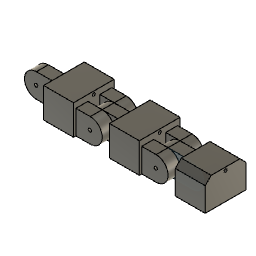
Complete Finger v1 (Autodesk Fusion 360 design; units mm, degrees)
Autodesk Fusion 360 part; units mm, degrees
sketch "Sketch3" plane through (0, 0, 0) normal (0, 1, 0) x (1, 0, 0)
  circle A0 centre (10, -10) radius 10
  circle A1 centre (-12.5, -10) radius 10
sketch "Sketch4" plane through (0, 0, 0) normal (0, 1, 0) x (1, 0, 0)
  line L0 (10, -20) -> (30, -20)
  line L1 (30, -20) -> (30, 0)
  line L2 (30, 0) -> (10, 0)
  line L3 (10, 0) -> (10, -20)
  circle A0 centre (30, -10) radius 10
  constraint horizontal L0
  constraint perpendicular L0 L1
  constraint perpendicular L1 L2
  constraint perpendicular L2 L3
  constraint midpoint L1 A0.centre
  constraint coincident L1.end A0
extrude "Extrude2" add sketch "Sketch4" sketch "Sketch3" along normal blind 10 of sketch 2 makes body 1 at (-2.5124, 6.6667, 10.4985) makes body 2 at (23.3333, 0, 13.3333)
sketch "Sketch5" plane through (0, 0, 0) normal (0, -1, 0) x (1, 0, 0)
  circle A0 centre (-12.5, 10) radius 10
  circle A1 centre (-12.5, 10) radius 10
  circle A2 centre (10, 10) radius 10
  line L0 (-12.5, 20) -> (10, 20)
  line L1 (10, 10) -> (10, 0)
  line L2 (-12.5, 0) -> (-12.5, 20)
  line L3 (10, 20) -> (10, 10)
  line L4 (-12.5, 0) -> (10, 0)
  constraint concentric A0 A1
  constraint coincident A1 L0.start
  constraint tangent A1 L0
  constraint horizontal L0
  constraint coincident A2.centre L1.start
  constraint coincident A2 L1.end
  constraint perpendicular L0 L1
  constraint coincident A1 L2.start
  constraint perpendicular L0 L2
  constraint perpendicular L0 L3
  constraint tangent A2 L4
extrude "Extrude3" add sketch "Sketch5" along normal blind 10 bodies 1 2
sketch "Sketch6" plane through (0, 10, 0) normal (0, 1, 0) x (-1, 0, 0)
  circle A0 centre (12.5, 10) radius 10
  circle A1 centre (12.5, 10) radius 10
  circle A2 centre (-10, 10) radius 10
  line L0 (-10, 20) -> (12.5, 20)
  line L1 (12.5, 10) -> (12.5, 0)
  line L2 (-10, 0) -> (-10, 10)
  line L3 (-10, 10) -> (-10, 20)
  line L4 (12.5, 10) -> (12.5, 20)
  line L5 (-10, 0) -> (12.5, 0)
  constraint concentric A0 A1
  constraint coincident A2 L0.start
  constraint coincident A1 L0.end
  constraint tangent A1 L0
  constraint horizontal L0
  constraint coincident A0.centre A1.centre
  constraint coincident A1 L1.end
  constraint perpendicular L0 L1
  constraint coincident A2 L2.start
  constraint coincident A2.centre L2.end
  constraint parallel L1 L2
  constraint perpendicular L0 L3
  constraint tangent A1 L5
extrude "Extrude4" add sketch "Sketch6" along normal blind 10 bodies 1
hole "Hole1" at (9.7334, -10, 10) direction (0, 1, 0) diameter 2.75 depth 38 tip angle 118 bodies 1
sketch "Sketch7" plane through (0, 0, 0) normal (0, -1, 0) x (1, 0, 0)
  arc A0 (10, 0) -> (10, 20) centre (10, 10) ccw
  line L0 (10, 0) -> (30, 0)
  arc A1 (30, 0) -> (30, 20) centre (30, 10) ccw
  line L1 (30, 20) -> (10, 20)
sketch "Sketch8" plane through (0, 0, 0) normal (0, 0, 1) x (1, 0, 0)
  line L0 (28, 10) -> (28, 22)
  line L1 (28, 22) -> (53, 22)
  line L2 (53, 22) -> (53, 0)
  line L3 (28, 0) -> (28, -12)
  line L4 (28, -12) -> (53, -12)
  line L5 (53, -12) -> (53, 0)
  line L6 (28, 10) -> (28, 0)
  constraint vertical L0
  constraint perpendicular L0 L1
  constraint perpendicular L1 L2
  constraint vertical L3
  constraint perpendicular L3 L4
  constraint perpendicular L4 L5
  constraint parallel L0 L6
extrude "Extrude5" add sketch "Sketch8" along normal blind 20 bodies 1
copy_body "CopyPasteBodies1" bodies 1 makes body 3
move_body "Move1" bodies 3 to x (1, 0, 0) y (0, 1, 0) z (0, 0, 1) at (-55, 0, 0)
copy_body "CopyPasteBodies2" bodies 1 makes body 4
move_body "Move2" bodies 4 to x (1, 0, 0) y (0, 1, 0) z (0, 0, 1) at (-110, 0, 0)
delete_face "DeleteFace1" 10 faces at (-107.5, 13.3333, 20) (-124.3925, 16.6667, 19.8193) (-123.4731, 3.3333, 0.0475) (-115.5459, -10, 10.0343) (-115, -3.3333, 20) (-97.5324, -6.6667, 0.3092) (-115.5459, 20, 10.0343) (-96.1157, 16.6667, 19.2148) (-107.5, 13.3333, 0) (-115, -3.3333, 0) on bodies 4
sketch "Sketch9" plane through (0, 0, 20) normal (0, 0, 1) x (-1, 0, 0)
  line L0 (82, -10) -> (100, -10)
  line L1 (100, -10) -> (100, 0)
  line L2 (100, 0) -> (82, 0)
  line L3 (82, 0) -> (82, 12)
  line L4 (82, 12) -> (57, 12)
  line L5 (57, 12) -> (57, -22)
  line L6 (57, -22) -> (82, -22)
  line L7 (82, -22) -> (82, -10)
  line L8 (57, 12) -> (57, 0)
  line L9 (57, -22) -> (82, -22)
  line L10 (82, 12) -> (57, 12)
  line L11 (82, 12) -> (82, -22)
  line L12 (57, -22) -> (57, 12)
  constraint coincident L4.end L5.start
  constraint coincident L5 L8.end
  constraint perpendicular L4 L8
  constraint coincident L5.end L6.start
  constraint coincident L6.end L7.start
  constraint coincident L3.end L4.start
extrude "Extrude6" add sketch "Sketch9" along normal blind 5 contours L3 L4 L5 L6 L7 L8 L9 L10 L11 L12 bodies 4 3
sketch "Sketch10" plane through (0, 0, 20) normal (0, 0, 1) x (-1, 0, 0)
  line L0 (27, -10) -> (45, -10)
  line L1 (45, -10) -> (45, 0)
  line L2 (45, 0) -> (27, 0)
  line L3 (27, 0) -> (27, 12)
  line L4 (27, 12) -> (2, 12)
  line L5 (2, 12) -> (2, -22)
  line L6 (2, -22) -> (27, -22)
  line L7 (27, -22) -> (27, -10)
  line L8 (2, 12) -> (2, -22)
  line L9 (27, -22) -> (27, 12)
  constraint coincident L4.end L5.start
  constraint coincident L5.end L6.start
  constraint coincident L6.end L7.start
  constraint coincident L3.end L4.start
extrude "Extrude7" add sketch "Sketch10" along normal blind 5 contours L3 L4 L5 L6 L7 L8 L9 bodies 4 1
sketch "Sketch11" plane through (0, 0, 20) normal (0, 0, 1) x (-1, 0, 0)
  line L0 (-28, -10) -> (-10, -10)
  line L1 (-10, -10) -> (-10, 0)
  line L2 (-10, 0) -> (-28, 0)
  line L3 (-28, 0) -> (-28, 12)
  line L4 (-28, 12) -> (-53, 12)
  line L5 (-53, 12) -> (-53, -22)
  line L6 (-53, -22) -> (-28, -22)
  line L7 (-28, -22) -> (-28, -10)
  line L8 (-53, 12) -> (-28, 12)
  line L9 (-28, -22) -> (-53, -22)
  line L10 (-53, 12) -> (-53, -22)
  line L11 (-28, 12) -> (-28, -22)
  constraint coincident L4.end L5.start
  constraint coincident L3.end L4.start
  constraint coincident L6.end L7.start
  constraint coincident L5.end L6.start
extrude "Extrude8" add sketch "Sketch11" along normal blind 5 contours L3 L4 L5 L6 L7 L8 L9 L10 L11 bodies 4
hole "Hole2" at (-82, 5, 22.5) direction (1, 0, 0) diameter 2.5 depth 170 tip angle 118 bodies 4
chamfer "Chamfer3" distance 5 angle 45 2 edges at (40.5, -12, 25) (40.5, 22, 25) on bodies 4
